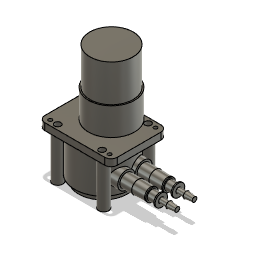
Peristaltic+Pump+(Rotated+Base) (Autodesk Fusion 360 design; units mm, degrees)
Autodesk Fusion 360 part; units mm, degrees
note: some values were not read from the file. Set by a fixed rule: which sketch regions a step uses.
sketch "Sketch1" plane through (0, 0, 0) normal (0, 1, 0) x (1, 0, 0)
  line L0 (29, 22.5) -> (-29, 22.5)
  line L1 (-29, 22.5) -> (-29, -22.5)
  line L2 (-29, -22.5) -> (29, -22.5)
  line L3 (29, -22.5) -> (29, 22.5)
  line L4 (29, 22.5) -> (-29, -22.5) construction
  line L5 (-29, 22.5) -> (29, -22.5) construction
  circle A0 centre (23.7156, -18.4) radius 1.45
  line L6 (0, -20) -> (0, -2.5)
  line L7 (2.5, 0) -> (20, 0)
  circle A1 centre (23.7156, 18.4) radius 1.45
  circle A2 centre (-23.7156, -18.4) radius 1.45
  circle A3 centre (-23.7156, 18.4) radius 1.45
  circle A4 centre (17.75, -18.4) radius 2.5
  circle A5 centre (17.75, 18.4) radius 2.5
  circle A6 centre (-17.75, 18.4) radius 2.5
  circle A7 centre (-17.75, -18.4) radius 2.5
  dimension "d1" = 58
  dimension "d2" = 45
  dimension "d3" = 2.9
  dimension "d4" = 4.1
  dimension "d5" = 5
  dimension "d6" = 4.1
  dimension "d7" = 17.75
  constraint perpendicular L0 L1
  constraint parallel L0 L2
  constraint parallel L1 L3
  constraint horizontal L0
  constraint coincident L4 origin
  constraint coincident L5 origin
  constraint coincident L5 A0.centre
  constraint symmetric A0 L7 A1
  constraint symmetric A0 L6 A2
  constraint symmetric L6 A1 A3
  constraint symmetric L7 A4 A5
  constraint symmetric L6 A4 A7
  constraint symmetric L6 A5 A6
  measures "d1" distance of L1.end L2.end
  measures "d2" distance of L0.start L2.end
  measures "d3" diameter of A0
  measures "d4" distance of L2 A0.centre
  measures "d5" diameter of A4
  measures "d6" distance of L2 A4.centre
  measures "d7" distance of L6 A4.centre
  measures "d21" diameter of L0.start
extrude "Extrude1" add sketch "Sketch1" along normal blind 5.5 makes body 1
sketch "Sketch2" plane through (0, 5.5, 0) normal (0, 1, 0) x (-1, 0, 0)
  circle A0 centre (17.75, 18.4) radius 2.5
  circle A1 centre (23.7156, -18.4) radius 1.45
  circle A2 centre (17.75, -18.4) radius 2.5
  circle A3 centre (-17.75, 18.4) radius 2.5
  circle A4 centre (-17.75, -18.4) radius 2.5
  circle A5 centre (-23.7156, -18.4) radius 1.45
  circle A6 centre (-23.7156, 18.4) radius 1.45
  circle A7 centre (23.7156, 18.4) radius 1.45
  line L0 (-29, 22.5) -> (-29, -22.5)
  line L1 (-29, -22.5) -> (29, -22.5)
  line L2 (29, -22.5) -> (29, 22.5)
  line L3 (29, 22.5) -> (-29, 22.5)
  circle A8 centre (0, -6.875) radius 18.375
  line L4 (0, 20) -> (0, 2.5)
  dimension "d10" = 36.75
  dimension "d11" = 29.375
  constraint coincident A8.centre L4
  measures "d10" diameter of A8
  measures "d11" distance of L3 A8.centre
extrude "Extrude2" add sketch "Sketch2" along normal blind 22 contours L1 A8 | L1 A8 bodies 1
sketch "Sketch3" plane through (0, 27.5, 0) normal (0, 1, 0) x (-1, 0, 0)
  circle A0 centre (0, -6.875) radius 17.3
  circle A1 centre (0, -6.875) radius 18.375
  dimension "d14" = 34.6
  constraint concentric A0 A1
  measures "d14" diameter of A0
extrude "Extrude3" add sketch "Sketch3" along normal blind 29.6 contours A0 bodies 1
sketch "Sketch4" plane through (0, 0, 0) normal (0, -1, 0) x (1, 0, 0)
  circle A0 centre (-17.75, 18.4) radius 2.5
  circle A1 centre (-23.7156, -18.4) radius 1.45
  circle A2 centre (-17.75, -18.4) radius 2.5
  circle A3 centre (17.75, 18.4) radius 2.5
  circle A4 centre (17.75, -18.4) radius 2.5
  circle A5 centre (23.7156, -18.4) radius 1.45
  circle A6 centre (23.7156, 18.4) radius 1.45
  circle A7 centre (-23.7156, 18.4) radius 1.45
  line L0 (29, -22.5) -> (29, 22.5)
  line L1 (29, 22.5) -> (-29, 22.5)
  line L2 (-29, 22.5) -> (-29, -22.5)
  line L3 (-29, -22.5) -> (29, -22.5)
  circle A8 centre (-17.75, 18.4) radius 4.1
  line L4 (0, 1.75) -> (0, 22.5)
  line L5 (1.75, 0) -> (22.5, 0)
  circle A9 centre (17.75, 18.4) radius 4.1
  circle A10 centre (-17.75, -18.4) radius 4.1
  circle A11 centre (17.75, -18.4) radius 4.1
  circle A12 centre (0, 0) radius 22.5
  constraint concentric A0 A8
  constraint tangent L1 A8
  constraint symmetric A8 L4 A9
  constraint symmetric A8 L5 A10
  constraint symmetric L5 A9 A11
  constraint coincident A12.centre origin
  constraint tangent L3 A12
extrude "Extrude4" add sketch "Sketch4" along normal blind 33.6 contours A11 A12 | A9 A12 | A8 A9 A10 A11 A12 | A11 A12 | A9 A12 | A10 A12 | A10 A12 | A8 A12 | A8 A12 bodies 1
sketch "Sketch5" plane through (0, -33.6, 0) normal (0, -1, 0) x (1, 0, 0)
  circle A0 centre (-17.75, -18.4) radius 2.5
  circle A1 centre (17.75, 18.4) radius 2.5
  circle A2 centre (-17.75, 18.4) radius 2.5
  circle A3 centre (17.75, -18.4) radius 2.5
  arc A4 (17.3556, -14.319) -> (17.3556, 14.319) centre (0, 0) ccw
  arc A5 (17.3556, 14.319) -> (13.6858, 17.8591) centre (17.75, 18.4) ccw
  arc A6 (13.6858, 17.8591) -> (-13.6858, 17.8591) centre (0, 0) ccw
  arc A7 (-13.6858, 17.8591) -> (-17.3556, 14.319) centre (-17.75, 18.4) ccw
  arc A8 (-17.3556, 14.319) -> (-17.3556, -14.319) centre (0, 0) ccw
  arc A9 (-17.3556, -14.319) -> (-13.6858, -17.8591) centre (-17.75, -18.4) ccw
  arc A10 (-13.6858, -17.8591) -> (13.6858, -17.8591) centre (0, 0) ccw
  arc A11 (13.6858, -17.8591) -> (17.3556, -14.319) centre (17.75, -18.4) ccw
  circle A12 centre (-17.75, 18.4) radius 4.1
  circle A13 centre (17.75, 18.4) radius 4.1
  circle A14 centre (17.75, -18.4) radius 4.1
  circle A15 centre (-17.75, -18.4) radius 4.1
  circle A16 centre (0, 0) radius 22.5
  line L0 (-18.2898, 17.8793) -> (-17.2102, 18.9207)
  line L1 (-17.2102, 18.9207) -> (18.2898, -17.8793)
  line L2 (18.2898, -17.8793) -> (17.2102, -18.9207)
  line L3 (17.2102, -18.9207) -> (-18.2898, 17.8793)
  line L4 (-18.2898, 17.8793) -> (18.2898, -17.8793) construction
  line L5 (-17.2102, 18.9207) -> (17.2102, -18.9207) construction
  line L6 (18.2898, 17.8793) -> (17.2102, 18.9207)
  line L7 (17.2102, 18.9207) -> (-18.2898, -17.8793)
  line L8 (-18.2898, -17.8793) -> (-17.2102, -18.9207)
  line L9 (-17.2102, -18.9207) -> (18.2898, 17.8793)
  line L10 (18.2898, 17.8793) -> (-18.2898, -17.8793) construction
  line L11 (17.2102, 18.9207) -> (-17.2102, -18.9207) construction
  circle A17 centre (0, 0) radius 19.375
  dimension "d20" = 1.5
  dimension "d21" = 8.2
  dimension "d22" = 8.2
  dimension "d23" = 8.2
  dimension "d24" = 45
  dimension "d25" = 1.5
  dimension "d26" = 38.75
  constraint concentric A2 A12
  constraint concentric A1 A13
  constraint concentric A3 A14
  constraint concentric A0 A15
  constraint concentric A4 A16
  constraint perpendicular L0 L1
  constraint parallel L0 L2
  constraint parallel L1 L3
  constraint coincident L4 A4.centre
  constraint coincident L5 A4.centre
  constraint coincident A4.centre A6.centre
  constraint midpoint A2.centre L0
  constraint perpendicular L6 L7
  constraint parallel L6 L8
  constraint parallel L7 L9
  constraint coincident L10 A4.centre
  constraint coincident L11 A4.centre
  constraint midpoint A1.centre L6
  constraint concentric A4 A17
  measures "d20" distance of L1 L3
  measures "d21" diameter of A15
  measures "d22" diameter of A12
  measures "d23" diameter of A13
  measures "d24" diameter of A16
  measures "d25" distance of L6.start L6.end
  measures "d26" diameter of A17
extrude "Extrude5" cut sketch "Sketch5" against normal blind 4.8 contours A10 A14 A15 A16 L3 L9 A17 | A8 A12 A15 A16 L3 L7 A17 | A4 A13 A14 A16 L1 L9 A17 | A6 A12 A13 A16 L1 L7 A17 bodies 1
sketch "Sketch6" plane through (0, -33.6, 0) normal (0, -1, 0) x (1, 0, 0)
  arc A0 (-14.4117, 16.0197) -> (-15.4913, 14.9783) centre (-17.75, 18.4) ccw
  line L0 (-15.4913, 14.9783) -> (-13.9814, 13.4131)
  arc A1 (-13.9814, 13.4131) -> (-13.9814, -13.4131) centre (0, 0) ccw
  line L1 (-13.9814, -13.4131) -> (-15.4913, -14.9783)
  arc A2 (-15.4913, -14.9783) -> (-14.4117, -16.0197) centre (-17.75, -18.4) ccw
  line L2 (-14.4117, -16.0197) -> (-12.9018, -14.4545)
  arc A3 (-12.9018, -14.4545) -> (12.9018, -14.4545) centre (0, 0) ccw
  line L3 (12.9018, -14.4545) -> (14.4117, -16.0197)
  arc A4 (14.4117, -16.0197) -> (15.4913, -14.9783) centre (17.75, -18.4) ccw
  line L4 (15.4913, -14.9783) -> (13.9814, -13.4131)
  arc A5 (13.9814, -13.4131) -> (13.9814, 13.4131) centre (0, 0) ccw
  line L5 (13.9814, 13.4131) -> (15.4913, 14.9783)
  arc A6 (15.4913, 14.9783) -> (14.4117, 16.0197) centre (17.75, 18.4) ccw
  line L6 (14.4117, 16.0197) -> (12.9018, 14.4545)
  arc A7 (12.9018, 14.4545) -> (-12.9018, 14.4545) centre (0, 0) ccw
  line L7 (-12.9018, 14.4545) -> (-14.4117, 16.0197)
  circle A8 centre (-17.75, -18.4) radius 2.5
  circle A9 centre (17.75, 18.4) radius 2.5
  circle A10 centre (-17.75, 18.4) radius 2.5
  circle A11 centre (17.75, -18.4) radius 2.5
  circle A12 centre (0, 0) radius 10.35
  circle A13 centre (0, 0) radius 6.35
  line L8 (-15.4913, 14.9783) -> (14.4117, -16.0197)
  line L9 (7.7067, -6.9087) -> (15.4913, -14.9783)
  line L10 (15.4913, 14.9783) -> (7.7067, 6.9087)
  line L11 (-13.9814, -13.4131) -> (14.4117, 16.0197)
  line L12 (-12.9018, -14.4545) -> (-6.3723, -8.1557)
  line L13 (-14.4117, 16.0197) -> (-6.6271, 7.9501)
  arc A14 (-14.4117, 16.0197) -> (-15.4913, 14.9783) centre (-17.75, 18.4) ccw
  arc A15 (15.4913, 14.9783) -> (14.4117, 16.0197) centre (17.75, 18.4) ccw
  arc A16 (14.4117, -16.0197) -> (15.4913, -14.9783) centre (17.75, -18.4) ccw
  arc A17 (-15.4913, -14.9783) -> (-14.4117, -16.0197) centre (-17.75, -18.4) ccw
  dimension "d29" = 20.7
  dimension "d30" = 4
  constraint coincident A1.centre A3.centre
  constraint concentric A12 A13
  constraint coincident A0.end L0.start
  constraint coincident L3.end A4.start
  constraint coincident A12 L9.start
  constraint coincident A4.end L4.start
  constraint parallel L4 L9
  constraint coincident L5.end A6.start
  constraint coincident A12 L10.end
  constraint coincident A1.end L1.start
  constraint coincident A6.end L6.start
  constraint parallel L10 L11
  constraint coincident L2.end A3.start
  constraint coincident A12 L12.end
  constraint perpendicular L8 L12
  constraint coincident A0.start L7.end
  constraint coincident A12 L13.end
  constraint parallel L7 L13
  measures "d29" diameter of A12
  measures "d30" distance of A12 A13
extrude "Extrude6" add sketch "Sketch6" along normal blind 1 contours A0 L0 L7 A12 L8 L13 A14 | L5 A6 L6 A12 L10 L11 A15 | A12 A13 L8 L11 | L1 A2 L2 A12 L11 L12 A17 | A12 A13 L8 L11 | A12 A13 L8 L11 | A12 A13 L8 L11 | L3 A4 L4 A12 L8 L9 A16 bodies 1
fillet "Fillet1" radius 5 4 edges at (29, 2.75, 22.5) (-29, 2.75, 22.5) (29, 2.75, -22.5) (-29, 2.75, -22.5) on bodies 1
ref_plane "WorkPlane1" through (0, -20.715, 22.5) normal (0, 0, 1) x (1, 0, 0)
ref_plane "WorkPlane2" through (0, -20.715, 25.7) normal (0, 0, 1) x (1, 0, 0)
sketch "Sketch7" plane through (0, -20.715, 25.7) normal (0, 0, 1) x (1, 0, 0)
  circle A0 centre (-6.9, 3.515) radius 6.9
  line L0 (-17.75, 20.715) -> (0, 20.715)
  line L1 (0, 23.215) -> (0, 40.715)
  circle A1 centre (6.9, 3.515) radius 6.9
  dimension "d36" = 13.8
  dimension "d37" = 17.2
  constraint tangent A0 L1
  constraint symmetric A0 L1 A1
  measures "d36" diameter of A0
  measures "d37" distance of A0.centre L0
extrude "Extrude7" add sketch "Sketch7" along normal up to surface end surface at (0, -19.2, 22.5) on bodies 1 bodies 1
sketch "Sketch8" plane through (0, 0, 25.7) normal (0, 0, 1) x (1, 0, 0)
  circle A0 centre (6.9, -17.2) radius 6.9
  line L0 (0, 2.5) -> (0, 20)
  circle A1 centre (-6.9, -17.2) radius 5.3
  circle A2 centre (-6.9, -17.2) radius 6.9
  circle A3 centre (6.9, -17.2) radius 5.3
  dimension "d40" = 10.6
  constraint concentric A1 A2
  constraint symmetric L0 A1 A3
  measures "d40" diameter of A1
extrude "Extrude8" add sketch "Sketch8" along normal blind 9.5 contours A1 | A3 bodies 1
ref_plane "WorkPlane3" through (-6.9, -17.2, 45.2) normal (0, 0, 1) x (1, 0, 0)
sketch "Sketch9" plane through (-6.9, -17.2, 45.2) normal (0, 0, 1) x (1, 0, 0)
  circle A0 centre (0, 0) radius 5
  circle A1 centre (13.8, 0) radius 5
  circle A2 centre (13.8, 0) radius 5.3
  dimension "d44" = 10
  dimension "d45" = 10
  constraint coincident A0.centre origin
  constraint concentric A1 A2
  measures "d44" diameter of A0
  measures "d45" diameter of A1
loft "Loft1" add profiles "Sketch9" section 1 contours A0 section 2 face at (-8.4917, -16.9251, 35.2) on bodies 1 bodies 1
loft "Loft2" add profiles "Sketch9" section 1 face at (8.0015, -15.2921, 35.2) section 2 contours A1 on bodies 1 bodies 1
extrude "Extrude9" add 2 faces at (-8.8305, -16.3446, 45.2) (4.9695, -16.3446, 45.2) along direction (0, 0, 1) blind 1 on bodies 1 bodies 1
sketch "Sketch10" plane through (0, 0, 46.2) normal (0, 0, 1) x (1, 0, 0)
  circle A0 centre (-6.9, -17.2) radius 5
  circle A1 centre (-6.9, -17.2) radius 3.875
  circle A2 centre (6.9, -17.2) radius 3.875
  circle A3 centre (6.9, -17.2) radius 5
  dimension "d48" = 7.75
  dimension "d49" = 7.75
  constraint concentric A0 A1
  constraint concentric A2 A3
  measures "d48" diameter of A1
  measures "d49" diameter of A2
extrude "Extrude10" add sketch "Sketch10" along normal blind 6.42 separate body contours A1 | A2 makes body 2 at (-3.0298, -17.3932, 50.48) makes body 3 at (10.7702, -17.3932, 50.48)
sketch "Sketch11" plane through (0, 0, 52.62) normal (0, 0, 1) x (1, 0, 0)
  circle A0 centre (-6.9, -17.2) radius 3.875
  circle A1 centre (-6.9, -17.2) radius 5
  circle A2 centre (6.9, -17.2) radius 5
  circle A3 centre (6.9, -17.2) radius 6.9
  dimension "d52" = 10
  dimension "d53" = 10
  constraint concentric A0 A1
  constraint concentric A2 A3
  measures "d52" diameter of A1
  measures "d53" diameter of A2
extrude "Extrude11" add sketch "Sketch11" along normal blind 1 contours A0 | A1 | A2 bodies 2 3
sketch "Sketch12" plane through (0, 0, 53.62) normal (0, 0, 1) x (1, 0, 0)
  circle A0 centre (-6.9, -17.2) radius 5
  circle A1 centre (-6.9, -17.2) radius 2.15
  circle A2 centre (6.9, -17.2) radius 2.15
  circle A3 centre (6.9, -17.2) radius 6.9
  dimension "d56" = 4.3
  dimension "d57" = 4.3
  constraint concentric A0 A1
  constraint concentric A2 A3
  measures "d56" diameter of A1
  measures "d57" diameter of A2
extrude "Extrude12" add sketch "Sketch12" along normal blind 6.32 contours A1 | A2 bodies 2 3
sketch "Sketch13" plane through (0, 0, 59.94) normal (0, 0, 1) x (1, 0, 0)
  circle A0 centre (-6.9, -17.2) radius 2.15
  circle A1 centre (-6.9, -17.2) radius 2.625
  circle A2 centre (6.9, -17.2) radius 2.625
  circle A3 centre (6.9, -17.2) radius 5
  dimension "d60" = 5.25
  dimension "d61" = 5.25
  constraint concentric A0 A1
  constraint concentric A2 A3
  measures "d60" diameter of A1
  measures "d61" diameter of A2
ref_plane "WorkPlane4" through (6.9, -17.2, 66.42) normal (0, 0, 1) x (1, 0, 0)
sketch "Sketch14" plane through (6.9, -17.2, 66.42) normal (0, 0, 1) x (1, 0, 0)
  circle A0 centre (0, 0) radius 1.875
  circle A1 centre (0, 0) radius 5
  circle A2 centre (-13.8, 0) radius 1.875
  circle A3 centre (-13.8, 0) radius 5
  dimension "d63" = 3.75
  dimension "d64" = 3.75
  constraint concentric A0 A1
  constraint concentric A2 A3
  measures "d63" diameter of A0
  measures "d64" diameter of A2
loft "Loft3" add profiles "Sketch13", "Sketch14" section 1 contours A0 | A1 section 2 contours A2 bodies 2
loft "Loft4" add profiles "Sketch13", "Sketch14" section 1 contours A2 section 2 contours A0 bodies 3
split "Split1" by plane through (0, 0, 0) normal (0, 1, 0) bodies 1 makes body 4 at (-17.214, 47.2333, -8.5975)
combine "Combine1" operation add target body 3 tool bodies 1
combine "Combine2" operation add target body 2 tool bodies 3
move_body "Move1" bodies 2 to x (0, 0, -1) y (0, 1, 0) z (1, 0, 0) at (0, 0, 0)
named bodies: "Peristaltic", "Motor and Mount"
